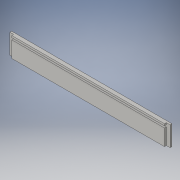
# Autodesk Inventor part: Base Runner Front
Saved by Autodesk Inventor 2016 (Build 200138000, 138)
## iProperties
Created: 2017-11-04
Part Number: Base Runner Front
Material: Generic
Document SubType Name: Modeling
Designer: mathaetaes
Density: 1 g/cm^3
Appearance: Default
Author: mathaetaes
Autodesk Inventor part; units mm, degrees
ref_plane "YZ Plane" through (0, 0, 0) normal (1, 0, 0) x (0, 1, 0)
ref_plane "XZ Plane" through (0, 0, 0) normal (0, 1, 0) x (-1, 0, 0)
ref_plane "XY Plane" through (0, 0, 0) normal (0, 0, 1) x (1, 0, 0)
sketch "Sketch2" plane through (0, 0, 0) normal (0, 0, 1) x (1, 0, 0)
  line L0 (-410.0497, 90.9112) -> (409.1003, 90.9112)
  line L1 (409.1003, 90.9112) -> (409.1003, -10.6888)
  line L2 (409.1003, -10.6888) -> (-410.0497, -10.6888)
  line L3 (-410.0497, -10.6888) -> (-410.0497, 90.9112)
  point P0 (0, 0)
  dimension "d0" = 819.15
  dimension "d1" = 101.6
  constraints: 8 end point, 2 parallel, 1 horizontal, 1 perpendicular
  measures "d0" distance of L0.start L0.end
  measures "d1" distance of L0.end L1.end
extrude "Board" add sketch "Sketch2" along normal blind 19.05
sketch "Sketch10" plane through (0, 0, 19.05) normal (0, 0, 1) x (1, 0, 0)
  line L0 (409.1003, -10.6888) -> (409.1003, 90.9112) projected
  line L1 (409.1003, 81.3862) -> (-410.0497, 81.3862)
  line L2 (-410.0497, 81.3862) -> (-410.0497, 71.8612)
  line L3 (-410.0497, 71.8612) -> (409.1003, 71.8612)
  line L4 (409.1003, 71.8612) -> (409.1003, 81.3862)
  line L5 (-410.0497, 90.9112) -> (-410.0497, -10.6888) projected
  line L6 (409.1003, 90.9112) -> (-410.0497, 90.9112) projected
  point P0 (0, 0)
  dimension "d22" = 9.525
  dimension "d23" = 9.525
  constraints: 8 end point, 2 parallel, 1 collinear, 1 horizontal, 1 perpendicular, 1 point on line
  measures "d22" distance between parallel lines of L1 L3
  measures "d23" distance between parallel lines of L6 L1
sketch "Sketch8" plane through (-410.0497, -10.6888, 0) normal (0, -1, 0) x (1, 0, 0)
  line L0 (819.15, 19.05) -> (0, 19.05) projected
  line L1 (0, 0) -> (0, 19.05) projected
  line L2 (0, 19.05) -> (0, 0)
  line L3 (0, 0) -> (19.05, 19.05)
  line L4 (19.05, 19.05) -> (0, 19.05)
  line L5 (819.15, 0) -> (819.15, 19.05) projected
  line L6 (819.15, 19.05) -> (819.15, 0)
  line L7 (819.15, 0) -> (800.1, 19.05)
  line L8 (800.1, 19.05) -> (819.15, 19.05)
  point P0 (410.0497, 0)
  dimension "d15" = 45
  dimension "d16" = 45
  constraints: 12 end point, 2 collinear, 2 point on line, 1 perpendicular, 1 vertical
  measures "d15" angle of L3 L2
  measures "d16" angle of L6 L7
extrude "45 degree mitre" [suppressed]
extrude "Extrusion7" cut sketch "Sketch10" against normal blind 9.525 contours L3 L2 L1 L0
sketch "Sketch11" plane through (-410.0497, 90.9112, 0) normal (0, 1, 0) x (1, 0, 0)
  line L0 (0, -19.05) -> (19.05, -19.05)
  line L1 (19.05, -19.05) -> (19.05, -9.525)
  line L2 (19.05, -9.525) -> (0, -9.525)
  line L3 (0, -9.525) -> (0, -19.05)
  line L4 (819.15, -9.525) -> (0, -9.525) projected
  line L5 (819.15, 0) -> (819.15, -19.05) projected
  line L6 (0, -9.525) -> (819.15, -9.525) projected
  line L7 (819.15, -19.05) -> (800.1, -19.05)
  line L8 (800.1, -19.05) -> (800.1, -9.525)
  line L9 (800.1, -9.525) -> (819.15, -9.525)
  line L10 (819.15, -9.525) -> (819.15, -19.05)
  point P0 (410.0497, 0)
  dimension "d28" = 19.05
  dimension "d29" = 19.05
  constraints: 16 end point, 4 parallel, 2 horizontal, 2 perpendicular, 1 collinear, 1 point on line
  measures "d28" distance between parallel lines of L1 L3
  measures "d29" distance of L8.end L9.end
extrude "End Notches" cut sketch "Sketch11" against normal blind 101.6
equation "\"d17\" = d1"
equation "\"d30\" = d1"
body "Solid1"
